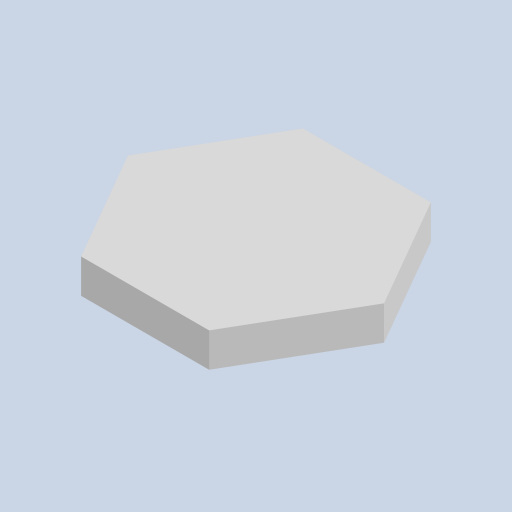
# Autodesk Inventor part: Capac_VarfBiti
Saved by Autodesk Inventor 2024 (Build 280153000, 153)
## iProperties
Created: 2024-04-20
Part Number: Capac_VarfBiti
Material: Generic
Document SubType Name: Modeling
Designer: mirun
Density: 1 g/cm^3
Appearance: Default
Author: mirun
Autodesk Inventor part; units mm, degrees
ref_plane "YZ Plane" through (0, 0, 0) normal (1, 0, 0) x (0, 1, 0)
ref_plane "XZ Plane" through (0, 0, 0) normal (0, 1, 0) x (-1, 0, 0)
ref_plane "XY Plane" through (0, 0, 0) normal (0, 0, 1) x (1, 0, 0)
sketch "Sketch1" plane through (0, 0, 0) normal (0, 1, 0) x (-1, 0, 0)
  line L0 (1.8764, 3.25) -> (3.7528, 0)
  line L1 (3.7528, 0) -> (1.8764, -3.25)
  line L2 (1.8764, -3.25) -> (-1.8764, -3.25)
  line L3 (-1.8764, -3.25) -> (-3.7528, 0)
  line L4 (-3.7528, 0) -> (-1.8764, 3.25)
  line L5 (-1.8764, 3.25) -> (1.8764, 3.25)
  circle A0 centre (0, 0) radius 2.5
  point P0 (0, 0)
  dimension "d0" = 6.5
  dimension "d1" = 5
  constraints: 12 end point, 1 centre point, 1 coincident, 13 other
  measures "d0" distance between parallel lines of L2 L5
  measures "d1" diameter of A0
extrude "Extrusion1" add sketch "Sketch1" along normal blind 1 contours L0 L1 L2 L3 L4 L5 | A0
extrude "Extrusion2" add sketch "Sketch1" against normal blind 0.35 contours A0
body "Solid1"
